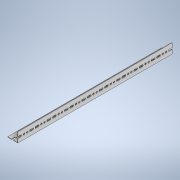
# Autodesk Inventor part: ChassisFrame
Saved by Autodesk Inventor 2020 (Build 240168000, 168)
## iProperties
Created: 2021-11-11
Part Number: ChassisFrame
Material: Generic
Document SubType Name: Modeling
Designer: 17185
Density: 1 g/cm^3
Appearance: Default
Author: 17185
Autodesk Inventor part; units mm, degrees
ref_plane "YZ Plane" through (0, 0, 0) normal (1, 0, 0) x (0, 1, 0)
ref_plane "XZ Plane" through (0, 0, 0) normal (0, 1, 0) x (-1, 0, 0)
ref_plane "XY Plane" through (0, 0, 0) normal (0, 0, 1) x (1, 0, 0)
sketch "Sketch1" plane through (0, 0, 0) normal (0, 1, 0) x (-1, 0, 0)
  line L0 (19.05, 304.8) -> (-19.05, 304.8)
  line L1 (-19.05, 304.8) -> (-19.05, -304.8)
  line L2 (-19.05, -304.8) -> (19.05, -304.8)
  line L3 (19.05, -304.8) -> (19.05, 304.8)
  line L4 (19.05, 304.8) -> (-19.05, -304.8) construction
  line L5 (-19.05, 304.8) -> (19.05, -304.8) construction
  circle A0 centre (0, 62.23) radius 3.556
  circle A1 centre (0, 6.35) radius 3.556
  line L6 (0, 304.8) -> (0, -304.8) construction
  line L7 (0, 49.53) -> (0, 40.64) construction
  line L8 (3.556, 49.53) -> (3.556, 40.64)
  line L9 (-3.556, 40.64) -> (-3.556, 49.53)
  arc A2 (3.556, 49.53) -> (-3.556, 49.53) centre (0, 49.53) ccw
  arc A3 (-3.556, 40.64) -> (3.556, 40.64) centre (0, 40.64) ccw
  line L10 (0, 27.94) -> (0, 19.05) construction
  line L11 (-3.556, 27.94) -> (-3.556, 19.05)
  line L12 (3.556, 19.05) -> (3.556, 27.94)
  arc A4 (3.556, 27.94) -> (-3.556, 27.94) centre (0, 27.94) ccw
  arc A5 (-3.556, 19.05) -> (3.556, 19.05) centre (0, 19.05) ccw
  line L13 (19.05, 68.58) -> (-6.1251, 68.58) construction
  line L14 (-6.1251, 68.58) -> (-19.05, 68.58) construction
  circle A6 centre (0, 74.93) radius 3.556
  circle A7 centre (0, 130.81) radius 3.556
  line L15 (0, 87.63) -> (0, 96.52) construction
  line L16 (3.556, 87.63) -> (3.556, 96.52)
  line L17 (-3.556, 96.52) -> (-3.556, 87.63)
  arc A8 (-3.556, 87.63) -> (3.556, 87.63) centre (0, 87.63) ccw
  arc A9 (3.556, 96.52) -> (-3.556, 96.52) centre (0, 96.52) ccw
  line L18 (0, 109.22) -> (0, 118.11) construction
  line L19 (-3.556, 109.22) -> (-3.556, 118.11)
  line L20 (3.556, 118.11) -> (3.556, 109.22)
  arc A10 (-3.556, 109.22) -> (3.556, 109.22) centre (0, 109.22) ccw
  arc A11 (3.556, 118.11) -> (-3.556, 118.11) centre (0, 118.11) ccw
  line L21 (19.05, 0) -> (-19.05, 0) construction
  circle A12 centre (0, -62.23) radius 3.556
  circle A13 centre (0, -6.35) radius 3.556
  line L22 (0, -49.53) -> (0, -40.64) construction
  line L23 (3.556, -49.53) -> (3.556, -40.64)
  line L24 (-3.556, -40.64) -> (-3.556, -49.53)
  arc A14 (-3.556, -49.53) -> (3.556, -49.53) centre (0, -49.53) ccw
  arc A15 (3.556, -40.64) -> (-3.556, -40.64) centre (0, -40.64) ccw
  line L25 (0, -27.94) -> (0, -19.05) construction
  line L26 (-3.556, -27.94) -> (-3.556, -19.05)
  line L27 (3.556, -19.05) -> (3.556, -27.94)
  arc A16 (-3.556, -27.94) -> (3.556, -27.94) centre (0, -27.94) ccw
  arc A17 (3.556, -19.05) -> (-3.556, -19.05) centre (0, -19.05) ccw
  line L28 (0, -109.22) -> (0, -118.11) construction
  line L29 (3.556, -118.11) -> (3.556, -109.22)
  arc A18 (3.556, -109.22) -> (-3.556, -109.22) centre (0, -109.22) ccw
  arc A19 (-3.556, -118.11) -> (3.556, -118.11) centre (0, -118.11) ccw
  circle A20 centre (0, -130.81) radius 3.556
  line L30 (-3.556, -109.22) -> (-3.556, -118.11)
  line L31 (0, -87.63) -> (0, -96.52) construction
  line L32 (-3.556, -96.52) -> (-3.556, -87.63)
  arc A21 (-3.556, -96.52) -> (3.556, -96.52) centre (0, -96.52) ccw
  arc A22 (3.556, -87.63) -> (-3.556, -87.63) centre (0, -87.63) ccw
  circle A23 centre (0, -74.93) radius 3.556
  line L33 (3.556, -87.63) -> (3.556, -96.52)
  line L34 (19.05, -137.16) -> (-19.05, -137.16) construction
  line L35 (19.05, 137.16) -> (-19.05, 137.16) construction
  circle A24 centre (0, 212.09) radius 3.556
  circle A25 centre (0, 267.97) radius 3.556
  line L36 (0, 224.79) -> (0, 233.68) construction
  line L37 (3.556, 224.79) -> (3.556, 233.68)
  line L38 (-3.556, 233.68) -> (-3.556, 224.79)
  arc A26 (-3.556, 224.79) -> (3.556, 224.79) centre (0, 224.79) ccw
  arc A27 (3.556, 233.68) -> (-3.556, 233.68) centre (0, 233.68) ccw
  line L39 (0, 246.38) -> (0, 255.27) construction
  line L40 (-3.556, 246.38) -> (-3.556, 255.27)
  line L41 (3.556, 255.27) -> (3.556, 246.38)
  arc A28 (-3.556, 246.38) -> (3.556, 246.38) centre (0, 246.38) ccw
  arc A29 (3.556, 255.27) -> (-3.556, 255.27) centre (0, 255.27) ccw
  line L42 (0, 165.1) -> (0, 156.21) construction
  line L43 (3.556, 156.21) -> (3.556, 165.1)
  arc A30 (3.556, 165.1) -> (-3.556, 165.1) centre (0, 165.1) ccw
  arc A31 (-3.556, 156.21) -> (3.556, 156.21) centre (0, 156.21) ccw
  circle A32 centre (0, 143.51) radius 3.556
  line L44 (-3.556, 165.1) -> (-3.556, 156.21)
  line L45 (0, 186.69) -> (0, 177.8) construction
  line L46 (-3.556, 177.8) -> (-3.556, 186.69)
  arc A33 (-3.556, 177.8) -> (3.556, 177.8) centre (0, 177.8) ccw
  arc A34 (3.556, 186.69) -> (-3.556, 186.69) centre (0, 186.69) ccw
  circle A35 centre (0, 199.39) radius 3.556
  line L47 (3.556, 186.69) -> (3.556, 177.8)
  arc A36 (3.556, 302.26) -> (-3.556, 302.26) centre (0, 302.26) ccw
  arc A37 (-3.556, 293.37) -> (3.556, 293.37) centre (0, 293.37) ccw
  circle A38 centre (0, 280.67) radius 3.556
  line L48 (-3.556, 302.26) -> (-3.556, 293.37)
  line L49 (3.556, 293.37) -> (3.556, 302.26)
  line L50 (0, 302.26) -> (0, 293.37) construction
  circle A39 centre (0, -280.67) radius 3.556
  line L51 (0, -302.26) -> (0, -293.37) construction
  line L52 (-3.556, -302.26) -> (-3.556, -293.37)
  line L53 (3.556, -293.37) -> (3.556, -302.26)
  arc A40 (-3.556, -302.26) -> (3.556, -302.26) centre (0, -302.26) ccw
  arc A41 (3.556, -293.37) -> (-3.556, -293.37) centre (0, -293.37) ccw
  line L54 (19.05, -274.32) -> (-19.05, -274.32) construction
  arc A42 (3.556, -246.38) -> (-3.556, -246.38) centre (0, -246.38) ccw
  arc A43 (-3.556, -255.27) -> (3.556, -255.27) centre (0, -255.27) ccw
  circle A44 centre (0, -267.97) radius 3.556
  line L55 (-3.556, -246.38) -> (-3.556, -255.27)
  line L56 (3.556, -255.27) -> (3.556, -246.38)
  line L57 (0, -246.38) -> (0, -255.27) construction
  line L58 (0, -224.79) -> (0, -233.68) construction
  line L59 (-3.556, -233.68) -> (-3.556, -224.79)
  circle A45 centre (0, -212.09) radius 3.556
  arc A46 (3.556, -224.79) -> (-3.556, -224.79) centre (0, -224.79) ccw
  line L60 (3.556, -224.79) -> (3.556, -233.68)
  arc A47 (-3.556, -233.68) -> (3.556, -233.68) centre (0, -233.68) ccw
  arc A48 (3.556, -177.8) -> (-3.556, -177.8) centre (0, -177.8) ccw
  arc A49 (-3.556, -165.1) -> (3.556, -165.1) centre (0, -165.1) ccw
  line L61 (0, -165.1) -> (0, -156.21) construction
  line L62 (-3.556, -165.1) -> (-3.556, -156.21)
  line L63 (3.556, -156.21) -> (3.556, -165.1)
  arc A50 (3.556, -156.21) -> (-3.556, -156.21) centre (0, -156.21) ccw
  circle A51 centre (0, -143.51) radius 3.556
  line L64 (0, -186.69) -> (0, -177.8) construction
  line L65 (-3.556, -177.8) -> (-3.556, -186.69)
  line L66 (3.556, -186.69) -> (3.556, -177.8)
  arc A52 (-3.556, -186.69) -> (3.556, -186.69) centre (0, -186.69) ccw
  circle A53 centre (0, -199.39) radius 3.556
  point P0 (0, 0)
  point P1 (0, 45.085)
  point P2 (0, 23.495)
  point P3 (0, 92.075)
  point P4 (0, 113.665)
  point P5 (0, -45.085)
  point P6 (0, -23.495)
  point P7 (-6.1251, -68.58)
  point P8 (0, -113.665)
  point P9 (0, -92.075)
  point P10 (0, 274.32)
  point P11 (0, 229.235)
  point P12 (0, 250.825)
  point P13 (-6.1251, 205.74)
  point P14 (0, 160.655)
  point P15 (0, 182.245)
  point P16 (0, 297.815)
  point P17 (0, -274.32)
  point P18 (0, -297.815)
  point P19 (0, -250.825)
  point P20 (0, -229.235)
  point P21 (0, -160.655)
  point P22 (-6.1251, -205.74)
  point P23 (0, -182.245)
  point P24 (2.4887, -304.8)
  point P25 (2.4887, 304.8)
  point P26 (-2.4887, 304.8)
  point P27 (-2.4887, -304.8)
  dimension "d1" = 609.6
  dimension "d3" = 7.112
  dimension "d6" = 7.112
  dimension "d9" = 3.556
  dimension "d10" = 3.556
  dimension "d11" = 6.35
  dimension "d12" = 12.7
  dimension "d13" = 8.89
  dimension "d14" = 8.89
  dimension "d15" = 12.7
  dimension "d16" = 12.7
  dimension "d26" = 6.35
  dimension "d29" = 6.35
  dimension "d30" = 6.35
  constraints: 170 end point, 135 symmetric about line, 72 point on circle, 54 centre point, 11 point on line, 8 midpoint, 8 tangent, 4 parallel, 3 perpendicular, 2 horizontal, 48 other
  measures "d1" distance of L0.end L1.end
  measures "d3" diameter of A1
  measures "d6" diameter of A0
  measures "d9" radius of A5
  measures "d10" radius of A3
  measures "d11" distance of A1.centre point (0, 0)
  measures "d12" distance of L10.end A1.centre
  measures "d13" distance of L10.start L10.end
  measures "d14" distance of L7.start L7.end
  measures "d15" distance of L10.start L7.end
  measures "d16" distance of L7.start A0.centre
  measures "d26" distance from line of A0.centre L13
  measures "d29" distance from line of L34 A20.centre
  measures "d30" distance from line of L35 A7.centre
extrude "Extrusion1" add sketch "Sketch1" along normal blind 1.9844 contours L3 L2 A40 L53 A41 L52 L1 L0 A36 L48 A37 L49
sketch "Sketch5" plane through (19.05, 0, 304.8) normal (1, 0, 0) x (0, 0, -1)
  line L0 (0.0028, 0.1675) -> (609.6028, 0.1675)
  line L1 (609.6028, 0.1675) -> (609.6028, 38.2675)
  line L2 (609.6028, 38.2675) -> (0.0028, 38.2675)
  line L3 (0.0028, 38.2675) -> (0.0028, 0.1675)
  line L4 (304.8, 0) -> (304.8028, 38.2675) construction
  line L5 (0.0028, 18.2448) -> (609.6028, 19.2175) construction
  circle A0 centre (298.4514, 18.721) radius 3.556
  line L6 (285.7514, 18.7007) -> (276.8614, 18.6866) construction
  line L7 (285.7457, 22.2567) -> (276.8557, 22.2426)
  line L8 (276.8671, 15.1306) -> (285.7571, 15.1448)
  arc A1 (285.7571, 15.1448) -> (285.7457, 22.2567) centre (285.7514, 18.7007) ccw
  arc A2 (276.8557, 22.2426) -> (276.8671, 15.1306) centre (276.8614, 18.6866) ccw
  line L9 (0, 0) -> (609.6, 0) construction
  line L10 (270.5114, 38.2675) -> (270.5114, 0) construction
  circle A3 centre (242.5714, 18.721) radius 3.556
  line L11 (255.2714, 18.7007) -> (264.1614, 18.6866) construction
  line L12 (255.2771, 22.2567) -> (264.1671, 22.2426)
  line L13 (264.1557, 15.1306) -> (255.2657, 15.1448)
  arc A4 (255.2771, 22.2567) -> (255.2657, 15.1448) centre (255.2714, 18.7007) ccw
  arc A5 (264.1557, 15.1306) -> (264.1671, 22.2426) centre (264.1614, 18.6866) ccw
  line L14 (236.2214, 38.2675) -> (236.2214, 0) construction
  circle A6 centre (173.9914, 18.721) radius 3.556
  line L15 (186.6914, 18.7007) -> (195.5814, 18.6866) construction
  line L16 (186.6971, 22.2567) -> (195.5871, 22.2426)
  line L17 (195.5757, 15.1306) -> (186.6858, 15.1448)
  arc A7 (186.6971, 22.2567) -> (186.6858, 15.1448) centre (186.6914, 18.7007) ccw
  arc A8 (195.5757, 15.1306) -> (195.5871, 22.2426) centre (195.5814, 18.6866) ccw
  line L18 (217.1714, 18.7007) -> (208.2814, 18.6866) construction
  line L19 (208.2871, 15.1306) -> (217.1771, 15.1448)
  arc A9 (208.2757, 22.2426) -> (208.2871, 15.1306) centre (208.2814, 18.6866) ccw
  circle A10 centre (229.8714, 18.721) radius 3.556
  arc A11 (217.1771, 15.1448) -> (217.1657, 22.2567) centre (217.1714, 18.7007) ccw
  line L20 (217.1657, 22.2567) -> (208.2757, 22.2426)
  line L21 (167.6414, 38.2675) -> (167.6414, 0) construction
  circle A12 centre (36.8315, 18.721) radius 3.556
  line L22 (49.5315, 18.7007) -> (58.4215, 18.6866) construction
  line L23 (49.5372, 22.2567) -> (58.4271, 22.2426)
  line L24 (58.4158, 15.1306) -> (49.5258, 15.1448)
  arc A13 (49.5372, 22.2567) -> (49.5258, 15.1448) centre (49.5315, 18.7007) ccw
  arc A14 (58.4158, 15.1306) -> (58.4271, 22.2426) centre (58.4215, 18.6866) ccw
  line L25 (80.0115, 18.7007) -> (71.1215, 18.6866) construction
  line L26 (71.1271, 15.1306) -> (80.0171, 15.1448)
  arc A15 (71.1158, 22.2426) -> (71.1271, 15.1306) centre (71.1215, 18.6866) ccw
  circle A16 centre (92.7115, 18.721) radius 3.556
  arc A17 (80.0171, 15.1448) -> (80.0058, 22.2567) centre (80.0115, 18.7007) ccw
  line L27 (80.0058, 22.2567) -> (71.1158, 22.2426)
  arc A18 (118.1171, 22.2567) -> (118.1058, 15.1448) centre (118.1115, 18.7007) ccw
  line L28 (118.1115, 18.7007) -> (127.0014, 18.6866) construction
  line L29 (118.1171, 22.2567) -> (127.0071, 22.2426)
  arc A19 (126.9958, 15.1306) -> (127.0071, 22.2426) centre (127.0014, 18.6866) ccw
  arc A20 (139.6958, 22.2426) -> (139.7071, 15.1306) centre (139.7014, 18.6866) ccw
  line L30 (148.5858, 22.2567) -> (139.6958, 22.2426)
  line L31 (139.7071, 15.1306) -> (148.5971, 15.1448)
  arc A21 (148.5971, 15.1448) -> (148.5858, 22.2567) centre (148.5914, 18.7007) ccw
  circle A22 centre (161.2914, 18.721) radius 3.556
  circle A23 centre (105.4115, 18.721) radius 3.556
  line L32 (148.5914, 18.7007) -> (139.7014, 18.6866) construction
  line L33 (126.9958, 15.1306) -> (118.1058, 15.1448)
  line L34 (30.4815, 38.2675) -> (30.4815, 0) construction
  arc A24 (11.4372, 15.1448) -> (11.4258, 22.2567) centre (11.4315, 18.7007) ccw
  line L35 (11.4315, 18.7007) -> (2.5415, 18.6866) construction
  line L36 (2.5472, 15.1306) -> (11.4372, 15.1448)
  arc A25 (2.5358, 22.2426) -> (2.5472, 15.1306) centre (2.5415, 18.6866) ccw
  circle A26 centre (24.1315, 18.721) radius 3.556
  line L37 (11.4258, 22.2567) -> (2.5358, 22.2426)
  circle A27 centre (311.1514, 18.7201) radius 3.556
  line L38 (323.8514, 18.6979) -> (332.7414, 18.6824) construction
  line L39 (323.8576, 22.2539) -> (332.7476, 22.2384)
  line L40 (332.7352, 15.1264) -> (323.8452, 15.1419)
  arc A28 (323.8576, 22.2539) -> (323.8452, 15.1419) centre (323.8514, 18.6979) ccw
  arc A29 (332.7352, 15.1264) -> (332.7476, 22.2384) centre (332.7414, 18.6824) ccw
  line L41 (354.3314, 18.6934) -> (345.4414, 18.6805) construction
  line L42 (345.4465, 15.1245) -> (354.3365, 15.1374)
  arc A30 (345.4362, 22.2365) -> (345.4465, 15.1245) centre (345.4414, 18.6805) ccw
  circle A31 centre (367.0314, 18.7118) radius 3.556
  arc A32 (354.3365, 15.1374) -> (354.3262, 22.2494) centre (354.3314, 18.6934) ccw
  line L43 (354.3262, 22.2494) -> (345.4362, 22.2365)
  arc A33 (392.4376, 22.2437) -> (392.4252, 15.1318) centre (392.4314, 18.6878) ccw
  line L44 (392.4314, 18.6878) -> (401.3213, 18.6722) construction
  line L45 (392.4376, 22.2437) -> (401.3275, 22.2282)
  arc A34 (401.3151, 15.1163) -> (401.3275, 22.2282) centre (401.3213, 18.6722) ccw
  arc A35 (414.0162, 22.2264) -> (414.0265, 15.1144) centre (414.0213, 18.6704) ccw
  line L46 (422.9062, 22.2392) -> (414.0162, 22.2264)
  line L47 (414.0265, 15.1144) -> (422.9165, 15.1272)
  arc A36 (422.9165, 15.1272) -> (422.9062, 22.2392) centre (422.9113, 18.6832) ccw
  circle A37 centre (435.6113, 18.7016) radius 3.556
  circle A38 centre (379.7314, 18.7099) radius 3.556
  line L48 (422.9113, 18.6832) -> (414.0213, 18.6704) construction
  line L49 (401.3151, 15.1163) -> (392.4252, 15.1318)
  arc A39 (560.0764, 15.1069) -> (560.0661, 22.2189) centre (560.0713, 18.6629) ccw
  line L50 (560.0713, 18.6629) -> (551.1813, 18.65) construction
  line L51 (551.1864, 15.094) -> (560.0764, 15.1069)
  arc A40 (551.1762, 22.206) -> (551.1864, 15.094) centre (551.1813, 18.65) ccw
  arc A41 (538.4751, 15.0959) -> (538.4875, 22.2079) centre (538.4813, 18.6519) ccw
  line L52 (529.5913, 18.6674) -> (538.4813, 18.6519) construction
  arc A42 (529.5975, 22.2234) -> (529.5851, 15.1114) centre (529.5913, 18.6674) ccw
  circle A43 centre (572.7713, 18.6813) radius 3.556
  line L53 (560.0661, 22.2189) -> (551.1762, 22.206)
  circle A44 centre (516.8913, 18.6896) radius 3.556
  line L54 (529.5975, 22.2234) -> (538.4875, 22.2079)
  line L55 (538.4751, 15.0959) -> (529.5851, 15.1114)
  circle A45 centre (504.1913, 18.6914) radius 3.556
  arc A46 (491.4965, 15.1171) -> (491.4862, 22.2291) centre (491.4913, 18.6731) ccw
  line L56 (491.4862, 22.2291) -> (482.5962, 22.2162)
  line L57 (491.4913, 18.6731) -> (482.6013, 18.6602) construction
  line L58 (482.6065, 15.1042) -> (491.4965, 15.1171)
  arc A47 (482.5962, 22.2162) -> (482.6065, 15.1042) centre (482.6013, 18.6602) ccw
  arc A48 (469.8951, 15.1061) -> (469.9075, 22.2181) centre (469.9013, 18.6621) ccw
  line L59 (461.0175, 22.2336) -> (469.9075, 22.2181)
  line L60 (461.0113, 18.6776) -> (469.9013, 18.6621) construction
  line L61 (469.8951, 15.1061) -> (461.0051, 15.1216)
  arc A49 (461.0175, 22.2336) -> (461.0051, 15.1216) centre (461.0113, 18.6776) ccw
  circle A50 centre (448.3113, 18.6997) radius 3.556
  arc A51 (598.1775, 22.2132) -> (598.1651, 15.1013) centre (598.1713, 18.6572) ccw
  line L62 (598.1713, 18.6572) -> (607.0613, 18.6417) construction
  line L63 (607.0551, 15.0857) -> (598.1651, 15.1013)
  arc A52 (607.0551, 15.0857) -> (607.0675, 22.1977) centre (607.0613, 18.6417) ccw
  line L64 (598.1775, 22.2132) -> (607.0675, 22.1977)
  circle A53 centre (585.4713, 18.6794) radius 3.556
  point P0 (281.3064, 18.6937)
  point P1 (259.7164, 18.6937)
  point P2 (191.1364, 18.6937)
  point P3 (212.7264, 18.6937)
  point P4 (53.9765, 18.6937)
  point P5 (75.5665, 18.6937)
  point P6 (122.5565, 18.6937)
  point P7 (144.1464, 18.6937)
  point P8 (6.9865, 18.6937)
  point P9 (609.5999, 18.1996)
  point P10 (328.2964, 18.6902)
  point P11 (349.8864, 18.687)
  point P12 (396.8764, 18.68)
  point P13 (418.4663, 18.6768)
  point P14 (555.6263, 18.6565)
  point P15 (534.0363, 18.6597)
  point P16 (487.0463, 18.6666)
  point P17 (465.4563, 18.6698)
  point P18 (602.6163, 18.6495)
  point P19 (609.6028, 21.1288)
  point P20 (0.0028, 21.1766)
  point P21 (0.0028, 16.1965)
  point P22 (609.6028, 16.1547)
  dimension "d61" = 609.6
  dimension "d62" = 38.1
  dimension "d63" = 7.112
  dimension "d64" = 8.89
  dimension "d65" = 7.112
  dimension "d66" = 6.35
  dimension "d67" = 12.7
  dimension "d72" = 6.35
  dimension "d73" = 6.35
  dimension "d74" = 6.35
  dimension "d75" = 6.35
  constraints: 164 end point, 137 symmetric about line, 72 point on circle, 54 centre point, 12 point on line, 4 tangent, 3 midpoint, 3 parallel, 3 perpendicular, 2 vertical, 1 horizontal, 51 other
  measures "d61" distance of L2.end L1.end
  measures "d62" distance of L0.end L1.end
  measures "d63" diameter of A0
  measures "d64" distance of L6.start L6.end
  measures "d65" diameter of A2
  measures "d66" distance from line of L4 A0.centre
  measures "d67" distance of A0.centre L6.start
  measures "d72" distance from line of L10 L6.end
  measures "d73" distance from line of L14 A3.centre
  measures "d74" distance from line of L21 A6.centre
  measures "d75" distance from line of L34 A12.centre
extrude "Extrusion2" add sketch "Sketch5" along normal blind 1.9844 contours L3 A25 L36 A24 L37 L2 L1 A52 L64 A51 L63 L0
equation "\"d6\" = d3"
equation "\"d9\" = 0.5 * d3"
equation "\"d10\" = d9"
equation "\"d14\" = d13"
equation "\"d15\" = d12"
equation "\"d16\" = d12"
equation "\"d65\" = d63"
equation "\"d72\" = d66"
equation "\"d73\" = d66"
equation "\"d74\" = d66"
equation "\"d75\" = d66"
body "Solid1"
